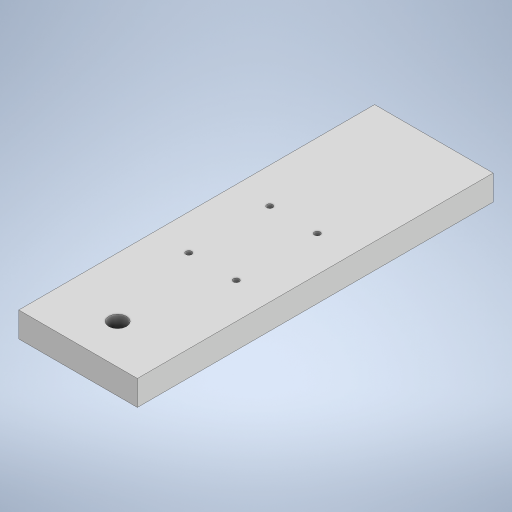
# Autodesk Inventor part: Carrier
Saved by Autodesk Inventor 2023 (Build 270158000, 158)
## iProperties
Created: 2023-03-15
Part Number: Carrier
Material: Generic
Document SubType Name: Modeling
Designer: Caleb
Density: 1 g/cm^3
Appearance: Default
Author: Caleb
Autodesk Inventor part; units mm, degrees
ref_plane "YZ Plane" through (0, 0, 0) normal (1, 0, 0) x (0, 1, 0)
ref_plane "XZ Plane" through (0, 0, 0) normal (0, 1, 0) x (-1, 0, 0)
ref_plane "XY Plane" through (0, 0, 0) normal (0, 0, 1) x (1, 0, 0)
sketch "Sketch1" plane through (0, 0, 0) normal (0, 1, 0) x (-1, 0, 0)
  line L0 (-15, -45) -> (15, -45)
  line L1 (15, -45) -> (15, 45)
  line L2 (15, 45) -> (-15, 45)
  line L3 (-15, 45) -> (-15, -45)
  line L4 (-15, -45) -> (15, 45) construction
  line L5 (15, -45) -> (-15, 45) construction
  point P0 (0, 0)
  dimension "d0" = 30
  dimension "d1" = 90
  constraints: 12 end point, 2 midpoint, 2 parallel, 1 horizontal, 1 perpendicular
  measures "d0" distance of L1.end L2.end
  measures "d1" distance of L0.end L1.end
extrude "Extrusion1" add sketch "Sketch1" along normal blind 6.35
sketch "Sketch2" plane through (0, 6.35, 0) normal (0, 1, 0) x (1, 0, 0)
  circle A0 centre (0, -35) radius 2.25
  line L0 (-15, -45) -> (15, -45) projected
  circle A1 centre (-6, -11) radius 0.75
  line L1 (-15, 45) -> (-15, -45) projected
  circle A2 centre (6, -11) radius 0.75
  circle A3 centre (-6, 9.5) radius 0.75
  circle A4 centre (6, 9.5) radius 0.75
  line L2 (15, -45) -> (15, 45) projected
  point P0 (0, 0)
  dimension "d4" = 4.5
  dimension "d5" = 10
  dimension "d6" = 34
  dimension "d7" = 9
  dimension "d8" = 1.5
  dimension "d9" = 1.5
  dimension "d10" = 1.5
  dimension "d11" = 1.5
  dimension "d12" = 9
  dimension "d13" = 20.5
  constraints: 5 centre point, 3 vertical alignment, 2 horizontal alignment
  measures "d4" diameter of A0
  measures "d5" distance from line of L0 A0.centre
  measures "d6" distance from line of L0 A1.centre
  measures "d7" distance from line of L1 A1.centre
  measures "d8" diameter of A1
  measures "d9" diameter of A2
  measures "d10" diameter of A3
  measures "d11" diameter of A4
  measures "d12" distance from line of A2.centre L2
  measures "d13" distance of A3.centre A1.centre
extrude "Extrusion2" cut sketch "Sketch2" against normal through all
equation "\"d9\" = d8"
equation "\"d10\" = d8"
equation "\"d11\" = d8"
equation "\"d12\" = d7"
body "Solid1"
